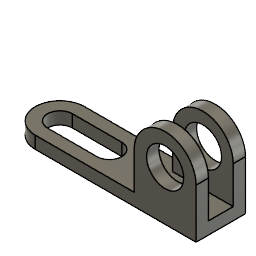
Exercise_5_Problem (Autodesk Fusion 360 design; units mm, degrees)
part number: 2026-05-18-23-19-58-246
Autodesk Fusion 360 part; units mm, degrees
note: some values were not read from the file. Set by a fixed rule: which sketch regions a step uses.
sketch "Sketch1" plane through (0, 0, 0) normal (0, 1, 0) x (1, 0, 0)
  line L0 (65, 20) -> (-65, 20)
  line L1 (-65, -20) -> (65, -20)
  line L2 (65, -20) -> (65, 20)
  line L3 (65, 20) -> (-65, -20) construction
  arc A0 (-65, 20) -> (-65, -20) centre (-65, 0) ccw
  arc A1 (-65, 10) -> (-65, -10) centre (-65, 0) ccw
  line L4 (-65, 20) -> (-25, 20)
  line L5 (-25, 10) -> (-65, 10)
  line L6 (-65, -10) -> (-25, -10)
  arc A2 (-25, -10) -> (-25, 10) centre (-25, 0) ccw
  line L7 (-65, 20) -> (-25, 7.6923) construction
  line L8 (-16.3592, 5.0336) -> (65, -20) construction
  line L9 (16, 20) -> (16, 10)
  line L10 (16, 10) -> (65, 10)
  line L11 (65, -20) -> (65, -10)
  line L12 (65, -10) -> (15, -10)
  line L13 (15, -10) -> (15, -20)
  dimension "d1" = 130
  dimension "d2" = 40
  dimension "d5" = 40
  dimension "d9" = 10
  dimension "d25" = 10
  dimension "d27" = 50
  constraint horizontal L0
  constraint parallel L0 L1
  constraint coincident L3 origin
  constraint coincident origin L8
  constraint concentric A0 A1
  constraint parallel L0 L4
  constraint tangent A1 L5
  constraint tangent L6 A2
  constraint parallel L5 L6
  constraint coincident A2 L8.start
  constraint collinear L7 L8
  constraint coincident L0 L9.start
  constraint perpendicular L0 L9
  constraint coincident L2 L10.end
  constraint perpendicular L2 L10
  constraint perpendicular L1 L11
  constraint perpendicular L2 L12
  constraint coincident L1 L13.end
  constraint perpendicular L1 L13
  measures "d1" distance of L1.start L1.end
  measures "d2" distance of L0.end L1.start
  measures "d5" distance of L0.end L4.end
  measures "d9" distance of L9.start L9.end
  measures "d25" distance of L1.end L11.end
  measures "d27" distance of L11.end L12.end
extrude "Extrude1" add sketch "Sketch1" along normal blind 10 contours L0 L1 L2 A0 L4 L9 L10 L12 L13
extrude "Extrude2" add sketch "Sketch1" along normal blind 65 contours L0 L2 L9 L10 | L1 L2 L11 L12 L13
sketch "Sketch2" plane through (0, 0, 20) normal (0, 0, 1) x (1, 0, 0)
  line L0 (-65, 0) -> (65, 0)
  line L1 (65, 0) -> (65, 65)
  line L2 (65, 65) -> (15, 65)
  line L3 (15, 10) -> (-65, 10)
  line L4 (-65, 10) -> (-65, 0)
  line L5 (65, 0) -> (65, 40)
  line L6 (65, 40) -> (40, 40)
  circle A0 centre (40, 40) radius 25
  circle A1 centre (40, 40) radius 15
  line L7 (15, 65) -> (15, 10)
  dimension "d16" = 40
  dimension "d17" = 30
  constraint coincident L0.end L1.start
  constraint perpendicular L0 L5
  constraint perpendicular L1 L6
  constraint coincident L6.end A0.centre
  constraint coincident L5.end A0
  constraint concentric A0 A1
  measures "d16" distance of L0.end L5.end
  measures "d17" diameter of A1
sketch "Sketch5" plane through (0, 0, -20) normal (0, 0, -1) x (-1, 0, 0)
  line L0 (-65, 0) -> (65, 0)
  line L1 (65, 0) -> (65, 10)
  line L2 (65, 10) -> (-16, 10)
  line L3 (-16, 10) -> (-16, 65)
  line L4 (-16, 65) -> (-65, 65)
  line L5 (-65, 65) -> (-65, 0)
  line L6 (-16, 10) -> (-16, 40)
  circle A0 centre (-40.5, 40) radius 24.5
  circle A1 centre (-40.5, 40) radius 15
  dimension "d29" = 30
  dimension "d30" = 30
  constraint coincident L2.end L3.start
  constraint perpendicular L2 L6
  constraint tangent L5 A0
  constraint coincident L6.end A0
  constraint concentric A0 A1
  measures "d29" distance of L2.end L6.end
  measures "d30" diameter of A1
extrude "Extrude5" cut sketch "Sketch5" against normal blind 10 contours L3 L4 L5 A0 | A1
extrude "Extrude6" cut sketch "Sketch2" against normal blind 10 contours L1 L2 A0 | L2 A0 L7 | A1
extrude "Extrude3" [rolled back] along distance -10 taper angle 0
extrude "Extrude4" [rolled back] along distance -10 taper angle 0
sketch "Sketch3" plane through (0, 0, -20) normal (0, 0, -1) x (-1, 0, 0)
  line L0 (-65, 0) -> (65, 0)
  line L1 (65, 0) -> (65, 10)
  line L2 (65, 10) -> (-16, 10)
  line L3 (-16, 10) -> (-16, 65)
  line L4 (-16, 65) -> (-65, 65)
  line L5 (-65, 65) -> (-65, 0)
  line L6 (-65, 0) -> (-65, 40)
  line L7 (-65, 40) -> (-40, 40)
  circle A0 centre (-40, 40) radius 25
  circle A1 centre (-40, 40) radius 15
  dimension "d22" = 40
  dimension "d23" = 50
  dimension "d24" = 30
  constraint coincident L0.start L5.end
  constraint perpendicular L0 L6
  constraint perpendicular L5 L7
  constraint coincident L7.end A0.centre
  constraint concentric A0 A1
  measures "d22" distance of L0.start L6.end
  measures "d23" diameter of A0
  measures "d24" diameter of A1
